Autodesk Inventor part; units mm, degrees
(part 2 of 2)
  spline S264 degree 2 poles (69.3218, -34.0148) (69.0307, -34.1828) (68.5047, -34.6064) (68.3514, -34.7463) knots 0 0 0 1 2 2 2
  line L285 (68.3514, -34.7463) -> (66.7794, -32.0236)
  line L286 (66.7794, -32.0236) -> (69.6777, -30.3503)
  line L287 (69.6777, -30.3503) -> (70.0361, -30.971)
  line L288 (70.0361, -30.971) -> (67.8185, -32.2513)
  line L289 (67.8185, -32.2513) -> (68.6317, -33.6598)
  spline S265 degree 2 poles (68.6317, -33.6598) (68.7502, -33.5685) (68.9911, -33.4123) (69.0938, -33.353) knots 0 0 0 1 2 2 2
  spline S266 degree 2 poles (69.0938, -33.353) (69.5005, -33.1182) (70.138, -32.9271) (70.5085, -32.9757) knots 0 0 0 1 2 2 2
  spline S267 degree 2 poles (70.5085, -32.9757) (70.8834, -33.0219) (71.5119, -33.4581) (71.7888, -33.9376) knots 0 0 0 1 2 2 2
  spline S268 degree 2 poles (75.2825, -30.6362) (76.103, -32.0575) (76.0455, -33.8659) (75.185, -34.3627) knots 0 0 0 1 2 2 2
  spline S269 degree 2 poles (75.185, -34.3627) (74.3117, -34.8669) (72.7105, -33.9819) (71.9072, -32.5906) knots 0 0 0 1 2 2 2
  spline S270 degree 2 poles (71.9072, -32.5906) (71.0817, -31.1607) (71.1442, -29.3609) (72.009, -28.8616) knots 0 0 0 1 2 2 2
  spline S271 degree 2 poles (72.009, -28.8616) (72.878, -28.3598) (74.4866, -29.2577) (75.2825, -30.6362) knots 0 0 0 1 2 2 2
  spline S272 degree 2 poles (75.3042, -32.7698) (75.2562, -32.4493) (74.8771, -31.5951) (74.5633, -31.0514) knots 0 0 0 1 2 2 2
  spline S273 degree 2 poles (74.5633, -31.0514) (74.2494, -30.5077) (73.7015, -29.7566) (73.4388, -29.5487) knots 0 0 0 1 2 2 2
  spline S274 degree 2 poles (73.4388, -29.5487) (73.1761, -29.3408) (72.643, -29.2775) (72.3476, -29.4481) knots 0 0 0 1 2 2 2
  spline S275 degree 2 poles (72.3476, -29.4481) (72.0522, -29.6186) (71.8318, -30.1169) (71.8812, -30.4594) knots 0 0 0 1 2 2 2
  spline S276 degree 2 poles (71.8812, -30.4594) (71.9299, -30.7909) (72.3274, -31.6573) (72.6264, -32.1753) knots 0 0 0 1 2 2 2
  spline S277 degree 2 poles (72.6264, -32.1753) (72.9477, -32.7319) (73.4463, -33.4372) (73.7257, -33.6641) knots 0 0 0 1 2 2 2
  spline S278 degree 2 poles (73.7257, -33.6641) (73.9866, -33.8787) (74.5382, -33.9541) (74.8464, -33.7762) knots 0 0 0 1 2 2 2
  spline S279 degree 2 poles (74.8464, -33.7762) (75.1375, -33.6081) (75.3579, -33.1099) (75.3042, -32.7698) knots 0 0 0 1 2 2 2
  spline S280 degree 2 poles (27.4559, -29.5461) (27.2633, -29.4349) (26.8279, -29.3091) (26.6018, -29.2756) knots 0 0 0 1 2 2 2
  spline S281 degree 2 poles (26.6018, -29.2756) (26.3885, -29.2495) (26.047, -29.2578) (25.909, -29.2695) knots 0 0 0 1 2 2 2
  line L290 (25.909, -29.2695) -> (25.8662, -29.2447)
  line L291 (25.8662, -29.2447) -> (26.2987, -28.4956)
  spline S282 degree 2 poles (26.2987, -28.4956) (26.6016, -28.5049) (27.5097, -28.7609) (27.865, -28.9661) knots 0 0 0 1 2 2 2
  spline S283 degree 2 poles (27.865, -28.9661) (28.2246, -29.1737) (28.6757, -29.6282) (28.8051, -29.9084) knots 0 0 0 1 2 2 2
  spline S284 degree 2 poles (28.8051, -29.9084) (28.9399, -30.2088) (28.9003, -30.831) (28.7124, -31.1563) knots 0 0 0 1 2 2 2
  spline S285 degree 2 poles (28.7124, -31.1563) (28.4603, -31.593) (27.5061, -31.9211) (27.0542, -31.7743) knots 0 0 0 1 2 2 2
  line L292 (27.0542, -31.7743) -> (27.0245, -31.8257)
  spline S286 degree 2 poles (27.0245, -31.8257) (27.1717, -31.9564) (27.4638, -32.3305) (27.5375, -32.5785) knots 0 0 0 1 2 2 2
  spline S287 degree 2 poles (27.5375, -32.5785) (27.6136, -32.8222) (27.5423, -33.4204) (27.3421, -33.7671) knots 0 0 0 1 2 2 2
  spline S288 degree 2 poles (27.3421, -33.7671) (27.137, -34.1224) (26.5444, -34.5852) (26.1884, -34.6878) knots 0 0 0 1 2 2 2
  spline S289 degree 2 poles (26.1884, -34.6878) (25.8188, -34.7941) (25.0204, -34.6642) (24.6052, -34.4245) knots 0 0 0 1 2 2 2
  spline S290 degree 2 poles (24.6052, -34.4245) (24.207, -34.1946) (23.5391, -33.5521) (23.3503, -33.2662) knots 0 0 0 1 2 2 2
  line L293 (23.3503, -33.2662) -> (23.7828, -32.517)
  line L294 (23.7828, -32.517) -> (23.8342, -32.5467)
  spline S291 degree 2 poles (23.8342, -32.5467) (23.9629, -32.8379) (24.5433, -33.5726) (24.9158, -33.7876) knots 0 0 0 1 2 2 2
  spline S292 degree 2 poles (24.9158, -33.7876) (25.1341, -33.9136) (25.6499, -34.0288) (25.8869, -33.9544) knots 0 0 0 1 2 2 2
  spline S293 degree 2 poles (25.8869, -33.9544) (26.1196, -33.8776) (26.4869, -33.5873) (26.6525, -33.3005) knots 0 0 0 1 2 2 2
  spline S294 degree 2 poles (26.6525, -33.3005) (26.8181, -33.0137) (26.8662, -32.5448) (26.7782, -32.3513) knots 0 0 0 1 2 2 2
  spline S295 degree 2 poles (26.7782, -32.3513) (26.6901, -32.1578) (26.3304, -31.8416) (26.0907, -31.7032) knots 0 0 0 1 2 2 2
  line L295 (26.0907, -31.7032) -> (25.791, -31.5302)
  line L296 (25.791, -31.5302) -> (26.1296, -30.9437)
  line L297 (26.1296, -30.9437) -> (26.3651, -31.0797)
  spline S296 degree 2 poles (26.3651, -31.0797) (26.8403, -31.354) (27.7016, -31.2462) (27.9512, -30.8139) knots 0 0 0 1 2 2 2
  spline S297 degree 2 poles (27.9512, -30.8139) (28.0674, -30.6127) (28.0789, -30.2369) (28.0042, -30.0796) knots 0 0 0 1 2 2 2
  spline S298 degree 2 poles (28.0042, -30.0796) (27.9234, -29.913) (27.64, -29.6524) (27.4559, -29.5461) knots 0 0 0 1 2 2 2
  spline S299 degree 2 poles (32.0466, -35.0505) (31.226, -36.4718) (29.6311, -37.3262) (28.7706, -36.8294) knots 0 0 0 1 2 2 2
  spline S300 degree 2 poles (28.7706, -36.8294) (27.8973, -36.3252) (27.8631, -34.496) (28.6664, -33.1047) knots 0 0 0 1 2 2 2
  spline S301 degree 2 poles (28.6664, -33.1047) (29.4919, -31.6748) (31.0819, -30.829) (31.9466, -31.3283) knots 0 0 0 1 2 2 2
  spline S302 degree 2 poles (31.9466, -31.3283) (32.8157, -31.83) (32.8424, -33.672) (32.0466, -35.0505) knots 0 0 0 1 2 2 2
  spline S303 degree 2 poles (30.2096, -36.1362) (30.4632, -35.9344) (31.0134, -35.179) (31.3273, -34.6353) knots 0 0 0 1 2 2 2
  spline S304 degree 2 poles (31.3273, -34.6353) (31.6412, -34.0916) (32.0178, -33.2416) (32.0665, -32.9101) knots 0 0 0 1 2 2 2
  spline S305 degree 2 poles (32.0665, -32.9101) (32.1152, -32.5786) (31.9034, -32.0853) (31.608, -31.9148) knots 0 0 0 1 2 2 2
  spline S306 degree 2 poles (31.608, -31.9148) (31.3126, -31.7443) (30.771, -31.8025) (30.499, -32.0165) knots 0 0 0 1 2 2 2
  spline S307 degree 2 poles (30.499, -32.0165) (30.2363, -32.2245) (29.6846, -33.0019) (29.3856, -33.5199) knots 0 0 0 1 2 2 2
  spline S308 degree 2 poles (29.3856, -33.5199) (29.0643, -34.0765) (28.7027, -34.8609) (28.6459, -35.2163) knots 0 0 0 1 2 2 2
  spline S309 degree 2 poles (28.6459, -35.2163) (28.5905, -35.5496) (28.801, -36.0649) (29.1092, -36.2429) knots 0 0 0 1 2 2 2
  spline S310 degree 2 poles (29.1092, -36.2429) (29.4003, -36.411) (29.942, -36.3527) (30.2096, -36.1362) knots 0 0 0 1 2 2 2
  spline S311 degree 2 poles (36.0108, -37.3393) (35.1902, -38.7606) (33.5953, -39.6149) (32.7348, -39.1181) knots 0 0 0 1 2 2 2
  spline S312 degree 2 poles (32.7348, -39.1181) (31.8615, -38.6139) (31.8273, -36.7848) (32.6306, -35.3934) knots 0 0 0 1 2 2 2
  spline S313 degree 2 poles (32.6306, -35.3934) (33.4561, -33.9636) (35.0461, -33.1178) (35.9108, -33.617) knots 0 0 0 1 2 2 2
  spline S314 degree 2 poles (35.9108, -33.617) (36.7799, -34.1188) (36.8066, -35.9608) (36.0108, -37.3393) knots 0 0 0 1 2 2 2
  spline S315 degree 2 poles (34.1739, -38.4249) (34.4274, -38.2231) (34.9777, -37.4677) (35.2916, -36.924) knots 0 0 0 1 2 2 2
  spline S316 degree 2 poles (35.2916, -36.924) (35.6054, -36.3803) (35.982, -35.5304) (36.0307, -35.1989) knots 0 0 0 1 2 2 2
  spline S317 degree 2 poles (36.0307, -35.1989) (36.0794, -34.8674) (35.8676, -34.3741) (35.5722, -34.2035) knots 0 0 0 1 2 2 2
  spline S318 degree 2 poles (35.5722, -34.2035) (35.2768, -34.033) (34.7352, -34.0913) (34.4632, -34.3053) knots 0 0 0 1 2 2 2
  spline S319 degree 2 poles (34.4632, -34.3053) (34.2005, -34.5132) (33.6489, -35.2907) (33.3498, -35.8087) knots 0 0 0 1 2 2 2
  spline S320 degree 2 poles (33.3498, -35.8087) (33.0285, -36.3652) (32.6669, -37.1496) (32.6101, -37.505) knots 0 0 0 1 2 2 2
  spline S321 degree 2 poles (32.6101, -37.505) (32.5547, -37.8383) (32.7652, -38.3537) (33.0734, -38.5316) knots 0 0 0 1 2 2 2
  spline S322 degree 2 poles (33.0734, -38.5316) (33.3645, -38.6997) (33.9062, -38.6414) (34.1739, -38.4249) knots 0 0 0 1 2 2 2
  line L298 (19.7742, -20.8876) -> (21.6551, -24.1454)
  line L299 (21.6551, -24.1454) -> (20.9059, -24.5779)
  spline S323 degree 2 poles (20.9059, -24.5779) (20.3736, -24.4172) (19.4006, -24.1456) (18.8979, -24.0363) knots 0 0 0 1 2 2 2
  spline S324 degree 2 poles (18.8979, -24.0363) (17.8859, -23.8158) (16.835, -23.8345) (16.4112, -24.0792) knots 0 0 0 1 2 2 2
  spline S325 degree 2 poles (16.4112, -24.0792) (16.1886, -24.2078) (15.9338, -24.5375) (15.8984, -24.7235) knots 0 0 0 1 2 2 2
  spline S326 degree 2 poles (15.8984, -24.7235) (15.8631, -24.9094) (15.9439, -25.2966) (16.0576, -25.4935) knots 0 0 0 1 2 2 2
  spline S327 degree 2 poles (16.0576, -25.4935) (16.1663, -25.6819) (16.483, -26.0128) (16.6571, -26.1463) knots 0 0 0 1 2 2 2
  spline S328 degree 2 poles (16.6571, -26.1463) (16.8035, -26.2615) (17.1354, -26.4409) (17.2448, -26.4919) knots 0 0 0 1 2 2 2
  line L300 (17.2448, -26.4919) -> (17.267, -26.5304)
  line L301 (17.267, -26.5304) -> (16.5136, -26.9655)
  spline S329 degree 2 poles (16.5136, -26.9655) (16.2805, -26.8089) (15.6184, -26.1466) (15.4157, -25.7956) knots 0 0 0 1 2 2 2
  spline S330 degree 2 poles (15.4157, -25.7956) (14.9881, -25.0549) (15.2896, -23.7678) (15.9574, -23.3823) knots 0 0 0 1 2 2 2
  spline S331 degree 2 poles (15.9574, -23.3823) (16.2699, -23.2018) (16.8763, -23.0459) (17.173, -23.0458) knots 0 0 0 1 2 2 2
  spline S332 degree 2 poles (17.173, -23.0458) (17.4783, -23.0407) (18.1472, -23.1512) (18.4841, -23.2306) knots 0 0 0 1 2 2 2
  spline S333 degree 2 poles (18.4841, -23.2306) (19.0408, -23.3544) (20.292, -23.7223) (20.6598, -23.8353) knots 0 0 0 1 2 2 2
  line L302 (20.6598, -23.8353) -> (19.162, -21.241)
  line L303 (19.162, -21.241) -> (19.7742, -20.8876)
  line L304 (15.5887, -17.8301) -> (15.9521, -18.4594)
  line L305 (15.9521, -18.4594) -> (17.7672, -17.4114)
  line L306 (17.7672, -17.4114) -> (18.1602, -18.0921)
  line L307 (18.1602, -18.0921) -> (16.345, -19.14)
  line L308 (16.345, -19.14) -> (17.6921, -21.4732)
  line L309 (17.6921, -21.4732) -> (16.9472, -21.9032)
  line L310 (16.9472, -21.9032) -> (12.8601, -21.1121)
  line L311 (12.8601, -21.1121) -> (12.4844, -20.4614)
  line L312 (12.4844, -20.4614) -> (15.3827, -18.7881)
  line L313 (15.3827, -18.7881) -> (15.0194, -18.1588)
  line L314 (15.0194, -18.1588) -> (15.5887, -17.8301)
  line L315 (15.7757, -19.4688) -> (13.7122, -20.6601)
  line L316 (13.7122, -20.6601) -> (16.8014, -21.2454)
  line L317 (16.8014, -21.2454) -> (15.7757, -19.4688)
  spline S334 degree 2 poles (12.538, -14.4542) (13.9593, -13.6336) (15.7677, -13.6911) (16.2645, -14.5516) knots 0 0 0 1 2 2 2
  spline S335 degree 2 poles (16.2645, -14.5516) (16.7687, -15.425) (15.8838, -17.0261) (14.4924, -17.8294) knots 0 0 0 1 2 2 2
  spline S336 degree 2 poles (14.4924, -17.8294) (13.0626, -18.6549) (11.2627, -18.5924) (10.7634, -17.7277) knots 0 0 0 1 2 2 2
  spline S337 degree 2 poles (10.7634, -17.7277) (10.2617, -16.8586) (11.1595, -15.25) (12.538, -14.4542) knots 0 0 0 1 2 2 2
  spline S338 degree 2 poles (14.6717, -14.4324) (14.3512, -14.4804) (13.4969, -14.8595) (12.9533, -15.1734) knots 0 0 0 1 2 2 2
  spline S339 degree 2 poles (12.9533, -15.1734) (12.4096, -15.4873) (11.6585, -16.0351) (11.4505, -16.2978) knots 0 0 0 1 2 2 2
  spline S340 degree 2 poles (11.4505, -16.2978) (11.2426, -16.5606) (11.1794, -17.0937) (11.3499, -17.3891) knots 0 0 0 1 2 2 2
  spline S341 degree 2 poles (11.3499, -17.3891) (11.5205, -17.6845) (12.0187, -17.9048) (12.3613, -17.8555) knots 0 0 0 1 2 2 2
  spline S342 degree 2 poles (12.3613, -17.8555) (12.6927, -17.8068) (13.5592, -17.4093) (14.0772, -17.1102) knots 0 0 0 1 2 2 2
  spline S343 degree 2 poles (14.0772, -17.1102) (14.6337, -16.7889) (15.3391, -16.2903) (15.5659, -16.011) knots 0 0 0 1 2 2 2
  spline S344 degree 2 poles (15.5659, -16.011) (15.7806, -15.75) (15.856, -15.1985) (15.678, -14.8902) knots 0 0 0 1 2 2 2
  spline S345 degree 2 poles (15.678, -14.8902) (15.51, -14.5991) (15.0117, -14.3788) (14.6717, -14.4324) knots 0 0 0 1 2 2 2
  line L318 (13.5615, -2.8735) -> (13.5615, -6.6353)
  line L319 (13.5615, -6.6353) -> (12.6964, -6.6353)
  spline S346 degree 2 poles (12.6964, -6.6353) (12.3158, -6.23) (11.6089, -5.5083) (11.2283, -5.1623) knots 0 0 0 1 2 2 2
  spline S347 degree 2 poles (11.2283, -5.1623) (10.4621, -4.4652) (9.5426, -3.9561) (9.0532, -3.9561) knots 0 0 0 1 2 2 2
  spline S348 degree 2 poles (9.0532, -3.9561) (8.7962, -3.9561) (8.4106, -4.1143) (8.287, -4.2576) knots 0 0 0 1 2 2 2
  spline S349 degree 2 poles (8.287, -4.2576) (8.1634, -4.401) (8.0398, -4.7767) (8.0398, -5.0041) knots 0 0 0 1 2 2 2
  spline S350 degree 2 poles (8.0398, -5.0041) (8.0398, -5.2216) (8.1486, -5.6665) (8.2326, -5.8691) knots 0 0 0 1 2 2 2
  spline S351 degree 2 poles (8.2326, -5.8691) (8.3018, -6.0422) (8.4996, -6.3635) (8.5688, -6.4623) knots 0 0 0 1 2 2 2
  line L320 (8.5688, -6.4623) -> (8.5688, -6.5068)
  line L321 (8.5688, -6.5068) -> (7.6988, -6.5068)
  spline S352 degree 2 poles (7.6988, -6.5068) (7.5752, -6.2547) (7.333, -5.3501) (7.333, -4.9447) knots 0 0 0 1 2 2 2
  spline S353 degree 2 poles (7.333, -4.9447) (7.333, -4.0896) (8.2376, -3.1256) (9.0087, -3.1256) knots 0 0 0 1 2 2 2
  spline S354 degree 2 poles (9.0087, -3.1256) (9.3696, -3.1256) (9.9727, -3.2937) (10.2297, -3.442) knots 0 0 0 1 2 2 2
  spline S355 degree 2 poles (10.2297, -3.442) (10.4967, -3.5903) (11.0206, -4.0204) (11.2727, -4.2576) knots 0 0 0 1 2 2 2
  spline S356 degree 2 poles (11.2727, -4.2576) (11.6929, -4.6432) (12.5926, -5.5874) (12.8546, -5.8691) knots 0 0 0 1 2 2 2
  line L322 (12.8546, -5.8691) -> (12.8546, -2.8735)
  line L323 (12.8546, -2.8735) -> (13.5615, -2.8735)
  line L324 (8.376, 1.7732) -> (13.5615, -0.8665)
  line L325 (13.5615, -0.8665) -> (13.5615, -1.7366)
  line L326 (13.5615, -1.7366) -> (8.1783, 1.0514)
  line L327 (8.1783, 1.0514) -> (8.1783, -2.0974)
  line L328 (8.1783, -2.0974) -> (7.4615, -2.0974)
  line L329 (7.4615, -2.0974) -> (7.4615, 1.7732)
  line L330 (7.4615, 1.7732) -> (8.376, 1.7732)
  spline S357 degree 2 poles (10.5115, 6.316) (12.1527, 6.316) (13.69, 5.362) (13.69, 4.3684) knots 0 0 0 1 2 2 2
  spline S358 degree 2 poles (13.69, 4.3684) (13.69, 3.36) (12.123, 2.4158) (10.5164, 2.4158) knots 0 0 0 1 2 2 2
  spline S359 degree 2 poles (10.5164, 2.4158) (8.8654, 2.4158) (7.3379, 3.3698) (7.3379, 4.3684) knots 0 0 0 1 2 2 2
  spline S360 degree 2 poles (7.3379, 4.3684) (7.3379, 5.3719) (8.9198, 6.316) (10.5115, 6.316) knots 0 0 0 1 2 2 2
  spline S361 degree 2 poles (12.3702, 5.2681) (12.0686, 5.3867) (11.1393, 5.4856) (10.5115, 5.4856) knots 0 0 0 1 2 2 2
  spline S362 degree 2 poles (10.5115, 5.4856) (9.8837, 5.4856) (8.9593, 5.3867) (8.6479, 5.2631) knots 0 0 0 1 2 2 2
  spline S363 degree 2 poles (8.6479, 5.2631) (8.3364, 5.1395) (8.0151, 4.7095) (8.0151, 4.3684) knots 0 0 0 1 2 2 2
  spline S364 degree 2 poles (8.0151, 4.3684) (8.0151, 4.0273) (8.3364, 3.5873) (8.6578, 3.4588) knots 0 0 0 1 2 2 2
  spline S365 degree 2 poles (8.6578, 3.4588) (8.9692, 3.3352) (9.9183, 3.2463) (10.5164, 3.2463) knots 0 0 0 1 2 2 2
  spline S366 degree 2 poles (10.5164, 3.2463) (11.1591, 3.2463) (12.0192, 3.3254) (12.3553, 3.4539) knots 0 0 0 1 2 2 2
  spline S367 degree 2 poles (12.3553, 3.4539) (12.6717, 3.5725) (13.0128, 4.0125) (13.0128, 4.3684) knots 0 0 0 1 2 2 2
  spline S368 degree 2 poles (13.0128, 4.3684) (13.0128, 4.7045) (12.6915, 5.1445) (12.3702, 5.2681) knots 0 0 0 1 2 2 2
  point P0 (0, 0)
  point P1 (97.5334, -46.673)
  point P2 (50, 21.5)
  point P3 (50, 35)
  point P4 (85.5155, 4.3292)
  point P5 (43.9223, 34.4683)
  point P6 (38.0293, 32.8892)
  point P7 (32.5, 30.3109)
  point P8 (27.5024, 26.8116)
  point P9 (23.1884, 22.4976)
  point P10 (19.6891, 17.5)
  point P11 (17.1108, 11.9707)
  point P12 (15.5317, 6.0777)
  point P13 (15, 0)
  point P14 (15.5317, -6.0777)
  point P15 (17.1108, -11.9707)
  point P16 (19.6891, -17.5)
  point P17 (23.1884, -22.4976)
  point P18 (27.5024, -26.8116)
  point P19 (32.5, -30.3109)
  point P20 (38.0293, -32.8892)
  point P21 (43.9223, -34.4683)
  point P22 (50, -35)
  point P23 (56.0777, -34.4683)
  point P24 (61.9707, -32.8892)
  point P25 (67.5, -30.3109)
  point P26 (72.4976, -26.8116)
  point P27 (76.8116, -22.4976)
  point P28 (80.3109, -17.5)
  point P29 (82.8892, -11.9707)
  point P30 (84.4683, -6.0777)
  point P31 (85, 0)
  point P32 (84.4683, 6.0777)
  point P33 (82.8892, 11.9707)
  point P34 (80.3109, 17.5)
  point P35 (76.8116, 22.4976)
  point P36 (72.4976, 26.8116)
  point P37 (67.5, 30.3109)
  point P38 (61.9707, 32.8892)
  point P39 (56.0777, 34.4683)
  point P40 (0, 15)
  point P41 (0, -15)
  point P42 (72.5, 38.9711)
  point P43 (72.5, -38.9711)
  point P44 (27.5, 38.9711)
  point P45 (27.5, -38.9711)
  point P46 (12.5, 24.8747)
  point P47 (12.5, -24.8747)
  dimension "d3" = 12
  dimension "d4" = 25
  dimension "d5" = 20.96
  dimension "d6" = 15.75
  dimension "d7" = 50
  dimension "d8" = 2.5
  dimension "d9" = 7
  dimension "d10" = 21.5
  dimension "d11" = 2.5
  dimension "d12" = 3
  dimension "d14" = 5
  dimension "d15" = 2
  dimension "d16" = 30
  dimension "d27" = 360
  dimension "d32" = 45
  dimension "d33" = 3
  dimension "d44" = 55
  dimension "d51" = 14.5786
  dimension "d52" = 14.5786
  dimension "d53" = 14.5786
  constraints: 320 end point, 30 point on circle, 20 centre point, 14 parallel, 8 point on line, 8 tangent, 7 equal radius, 6 midpoint, 6 perpendicular, 4 coincident, 4 horizontal, 2 concentric, 1 vertical, 360 other
  measures "d3" diameter of A0
  measures "d4" diameter of A1
  measures "d5" distance of A5.centre A4.centre
  measures "d6" distance from line of L1 A4.centre
  measures "d7" distance from line of L0 A0.centre
  measures "d8" radius of A3
  measures "d9" distance of L2.start L2.end
  measures "d10" distance from line of L1 L2.start
  measures "d11" diameter of A4
  measures "d12" diameter of A7
  measures "d14" distance of L12.end L10.start
  measures "d15" distance of L10.start L10.end
  measures "d16" distance from line of A0.centre L12
  measures "d32" radius of A11
  measures "d33" diameter of A13
  measures "d44" distance of L171.start L171.end
  measures "d51" distance of L189.end L190.end
  measures "d52" distance of L194.end L195.end
  measures "d53" distance of L198.end L199.end
extrude "Extrusion1" add sketch "Sketch1" against normal blind 4 contours L13 L12 L11 L10 | L34 L33 L32 L31 | L38 L37 L36 L35 | L42 L41 L40 L39 | L46 L45 L176 L43 | L43 L176 A19 S127 S126 S125 S124 S123 S122 S121 S120 A10 A18 S190 S189 S188 S187 L175 L157 L158 L155 L117 L118 L115 A16 S270 S269 S268 A11 A17 S290 S289 S288 S287 S286 L292 S285 S284 S283 L85 L86 L83 L45 L46 | L176 L45 L44 L43 | L43 L44 L45 L176 L83 L84 L85 A17 S283 S282 L291 L290 S281 S280 S298 S297 S296 L297 L296 L295 S295 S291 L294 L293 S290 A11 A10 A19 S120 L232 L231 S119 S118 S134 L238 L237 L236 S133 S132 S131 S130 S129 L235 L234 S128 S127 | S127 S128 L234 L235 S129 S130 S131 S132 S133 L236 L237 L238 S134 A19 S123 L233 S124 | A19 S124 S125 S126 S127 | L176 L85 L84 L83 | L83 L86 L85 L176 | S124 L233 S123 A19 | A19 S134 S135 S136 S118 S120 S121 S122 S123 | A19 S118 S136 S135 S134 | S283 S284 S285 L292 S286 S287 S288 S289 S290 A17 S291 S292 S293 S294 S295 S296 S297 | A17 S297 S298 S280 S281 L290 L291 S282 S283 | S118 S119 L231 L232 S120 A19 | S297 S296 A17 | A17 S295 L295 L296 L297 S296 | S295 S294 S293 S292 S291 A17 | A10 A11 A16 S268 S271 S270 L175 L115 L116 L117 L155 L156 L157 A18 S187 S190 | A17 S290 L293 L294 S291 | S190 S187 A18 S191 | A18 S191 S192 S193 S194 S195 S196 S197 S198 S187 S188 S189 S190 | S191 A18 | A18 S191 S198 S197 S196 S195 S194 S193 S192 | S268 S269 S270 A16 S275 S276 S277 S278 S279 | A16 S279 S272 S273 S274 S275 S270 S271 S268 | S279 S278 S277 S276 S275 A16 | A16 S275 S274 S273 S272 S279 | L175 L155 L158 L157 | L157 L156 L155 L175 | L175 L115 L118 L117 | L117 L116 L115 L175 | L50 L49 L48 L47 | L54 L53 L52 L51 | L58 L57 L56 L55 | L62 L61 L60 L59 | L66 L65 L64 L63 | L70 L69 L68 L67 | L74 L73 L72 L71 | L78 L77 L76 L75 | L82 L81 L80 L79 | L90 L89 L88 L87 | L94 L93 L92 L91 | L98 L97 L96 L95 | L102 L101 L100 L99 | L106 L105 L104 L103 | L110 L109 L108 L107 | L114 L113 L112 L111 | L122 L121 L120 L119 | L126 L125 L124 L123 | L130 L129 L128 L127 | L134 L133 L132 L131 | L138 L137 L136 L135 | L142 L141 L140 L139 | L146 L145 L144 L143 | L150 L149 L148 L147 | L154 L153 L152 L151 | L162 L161 L160 L159 | L166 L165 L164 L163 | L170 L169 L168 L167 | S0 S1 L209 L210 S2 S3 S4 S5 L211 S6 S7 S8 S9 S10 L212 L213 S11 S12 S13 S14 S15 L214 L215 L216 S16 S17 S18 | S19 S20 S21 S22 | S30 S29 S28 S27 S26 S25 S24 S23 | S31 S32 S33 S34 | S42 S41 S40 S39 S38 S37 S36 S35 | L217 L218 L219 L220 L221 L222 S43 L223 L224 L225 L226 | S44 S45 S46 L227 S47 S48 S49 S50 L228 S51 S52 | S57 S56 S55 S54 S53 | S62 S61 S60 S59 S58 | S63 S64 S65 S66 | S74 S73 S72 S71 S70 S69 S68 S67 | S75 S76 S77 S78 S79 S80 S81 L229 L230 S82 S83 S84 S85 S86 | S93 S92 S91 S90 S89 S88 S87 | S94 S95 S96 S97 | S105 S104 S103 S102 S101 S100 S99 S98 | S106 S107 S108 S109 | S117 S116 S115 S114 S113 S112 S111 S110 | S137 S138 L239 L240 S139 S140 S141 S142 L241 S143 S144 S145 S146 S147 L242 L243 S148 S149 S150 S151 S152 L244 L245 L246 S153 S154 S155 | S156 S157 S158 S159 | S167 S166 S165 S164 S163 S162 S161 S160 | S168 S169 L247 L248 S170 S171 S172 S173 L249 S174 S175 S176 S177 S178 L250 L251 S179 S180 S181 S182 S183 L252 L253 L254 S184 S185 S186 | S199 S200 S201 S202 S203 S204 S205 L255 L256 S206 S207 S208 S209 S210 | S217 S216 S215 S214 S213 S212 S211 | S218 S219 S220 S221 | S229 S228 S227 S226 S225 S224 S223 S222 | L257 L258 L259 L260 L261 L262 S230 L263 L264 L265 L266 | L267 L268 S231 S232 S233 S234 S235 S236 L269 L270 S237 S238 S239 S240 S241 L271 L272 | S242 S243 S244 S245 | S253 S252 S251 S250 S249 S248 S247 S246 | L273 L274 L275 L276 L277 L278 S254 L279 L280 L281 L282 | S255 S256 S257 L283 L284 S258 S259 S260 S261 S262 S263 S264 L285 L286 L287 L288 L289 S265 S266 S267 | S299 S300 S301 S302 | S310 S309 S308 S307 S306 S305 S304 S303 | S311 S312 S313 S314 | S322 S321 S320 S319 S318 S317 S316 S315 | L298 L299 S323 S324 S325 S326 S327 S328 L300 L301 S329 S330 S331 S332 S333 L302 L303 | L304 L305 L306 L307 L308 L309 L310 L311 L312 L313 L314 | L317 L316 L315 | S334 S335 S336 S337 | S345 S344 S343 S342 S341 S340 S339 S338 | L318 L319 S346 S347 S348 S349 S350 S351 L320 L321 S352 S353 S354 S355 S356 L322 L323 | L324 L325 L326 L327 L328 L329 L330 | S357 S358 S359 S360 | S368 S367 S366 S365 S364 S363 S362 S361
extrude "Extrusion2" add sketch "Sketch1" along normal blind 1.5 contours L13 L12 L11 L10 | L34 L33 L32 L31 | L38 L37 L36 L35 | L42 L41 L40 L39 | L46 L45 L176 L43 | L176 L45 L44 L43 | L176 L85 L84 L83 | L83 L86 L85 L176 | L175 L155 L158 L157 | L157 L156 L155 L175 | L175 L115 L118 L117 | L117 L116 L115 L175 | L50 L49 L48 L47 | L54 L53 L52 L51 | L58 L57 L56 L55 | L62 L61 L60 L59 | L66 L65 L64 L63 | L70 L69 L68 L67 | L74 L73 L72 L71 | L78 L77 L76 L75 | L82 L81 L80 L79 | L90 L89 L88 L87 | L94 L93 L92 L91 | L98 L97 L96 L95 | L102 L101 L100 L99 | L106 L105 L104 L103 | L110 L109 L108 L107 | L114 L113 L112 L111 | L122 L121 L120 L119 | L126 L125 L124 L123 | L130 L129 L128 L127 | L134 L133 L132 L131 | L138 L137 L136 L135 | L142 L141 L140 L139 | L146 L145 L144 L143 | L150 L149 L148 L147 | L154 L153 L152 L151 | L162 L161 L160 L159 | L166 L165 L164 L163 | L170 L169 L168 L167
extrude "Extrusion3" add sketch "Sketch1" along normal blind 1 contours S127 S128 L234 L235 S129 S130 S131 S132 S133 L236 L237 L238 S134 A19 S123 L233 S124 | A19 S124 S125 S126 S127 | A19 S134 S135 S136 S118 S120 S121 S122 S123 | S283 S284 S285 L292 S286 S287 S288 S289 S290 A17 S291 S292 S293 S294 S295 S296 S297 | A17 S297 S298 S280 S281 L290 L291 S282 S283 | S118 S119 L231 L232 S120 A19 | A17 S295 L295 L296 L297 S296 | A17 S290 L293 L294 S291 | S190 S187 A18 S191 | A18 S191 S192 S193 S194 S195 S196 S197 S198 S187 S188 S189 S190 | S268 S269 S270 A16 S275 S276 S277 S278 S279 | A16 S279 S272 S273 S274 S275 S270 S271 S268 | S0 S1 L209 L210 S2 S3 S4 S5 L211 S6 S7 S8 S9 S10 L212 L213 S11 S12 S13 S14 S15 L214 L215 L216 S16 S17 S18 | S19 S20 S21 S22 | S31 S32 S33 S34 | L217 L218 L219 L220 L221 L222 S43 L223 L224 L225 L226 | S44 S45 S46 L227 S47 S48 S49 S50 L228 S51 S52 | S63 S64 S65 S66 | S75 S76 S77 S78 S79 S80 S81 L229 L230 S82 S83 S84 S85 S86 | S94 S95 S96 S97 | S106 S107 S108 S109 | S137 S138 L239 L240 S139 S140 S141 S142 L241 S143 S144 S145 S146 S147 L242 L243 S148 S149 S150 S151 S152 L244 L245 L246 S153 S154 S155 | S156 S157 S158 S159 | S168 S169 L247 L248 S170 S171 S172 S173 L249 S174 S175 S176 S177 S178 L250 L251 S179 S180 S181 S182 S183 L252 L253 L254 S184 S185 S186 | S199 S200 S201 S202 S203 S204 S205 L255 L256 S206 S207 S208 S209 S210 | S218 S219 S220 S221 | L257 L258 L259 L260 L261 L262 S230 L263 L264 L265 L266 | L267 L268 S231 S232 S233 S234 S235 S236 L269 L270 S237 S238 S239 S240 S241 L271 L272 | S242 S243 S244 S245 | L273 L274 L275 L276 L277 L278 S254 L279 L280 L281 L282 | S255 S256 S257 L283 L284 S258 S259 S260 S261 S262 S263 S264 L285 L286 L287 L288 L289 S265 S266 S267 | S299 S300 S301 S302 | S311 S312 S313 S314 | L298 L299 S323 S324 S325 S326 S327 S328 L300 L301 S329 S330 S331 S332 S333 L302 L303 | L304 L305 L306 L307 L308 L309 L310 L311 L312 L313 L314 | S334 S335 S336 S337 | L318 L319 S346 S347 S348 S349 S350 S351 L320 L321 S352 S353 S354 S355 S356 L322 L323 | L324 L325 L326 L327 L328 L329 L330 | S357 S358 S359 S360
extrude "Extrusion4" add sketch "Sketch1" against normal blind 20 from surface at -4 separate body contours L176 L45 L44 L43 | L43 L44 L45 L176 L83 L84 L85 A17 S283 S282 L291 L290 S281 S280 S298 S297 S296 L297 L296 L295 S295 S291 L294 L293 S290 A11 A10 A19 S120 L232 L231 S119 S118 S134 L238 L237 L236 S133 S132 S131 S130 S129 L235 L234 S128 S127 | S127 S128 L234 L235 S129 S130 S131 S132 S133 L236 L237 L238 S134 A19 S123 L233 S124 | L176 L85 L84 L83 | S124 L233 S123 A19 | A17 S297 S298 S280 S281 L290 L291 S282 S283 | S118 S119 L231 L232 S120 A19 | A17 S295 L295 L296 L297 S296 | A10 A11 A16 S268 S271 S270 L175 L115 L116 L117 L155 L156 L157 A18 S187 S190 | A17 S290 L293 L294 S291 | S190 S187 A18 S191 | S191 A18 | A16 S279 S272 S273 S274 S275 S270 S271 S268 | A16 S275 S274 S273 S272 S279 | L157 L156 L155 L175 | L117 L116 L115 L175 | L50 L49 L48 L47 | L54 L53 L52 L51 | L58 L57 L56 L55 | L62 L61 L60 L59 | L66 L65 L64 L63 | L70 L69 L68 L67 | L74 L73 L72 L71 | L78 L77 L76 L75 | L82 L81 L80 L79 | L122 L121 L120 L119 | L126 L125 L124 L123 | L130 L129 L128 L127 | L134 L133 L132 L131 | L138 L137 L136 L135 | L142 L141 L140 L139 | L146 L145 L144 L143 | L150 L149 L148 L147 | L154 L153 L152 L151 | S0 S1 L209 L210 S2 S3 S4 S5 L211 S6 S7 S8 S9 S10 L212 L213 S11 S12 S13 S14 S15 L214 L215 L216 S16 S17 S18 | S19 S20 S21 S22 | S30 S29 S28 S27 S26 S25 S24 S23 | S31 S32 S33 S34 | S42 S41 S40 S39 S38 S37 S36 S35 | S75 S76 S77 S78 S79 S80 S81 L229 L230 S82 S83 S84 S85 S86 | S93 S92 S91 S90 S89 S88 S87 | S94 S95 S96 S97 | S105 S104 S103 S102 S101 S100 S99 S98 | S199 S200 S201 S202 S203 S204 S205 L255 L256 S206 S207 S208 S209 S210 | S217 S216 S215 S214 S213 S212 S211 | S218 S219 S220 S221 | S229 S228 S227 S226 S225 S224 S223 S222 | L257 L258 L259 L260 L261 L262 S230 L263 L264 L265 L266 | L267 L268 S231 S232 S233 S234 S235 S236 L269 L270 S237 S238 S239 S240 S241 L271 L272 | S242 S243 S244 S245 | S253 S252 S251 S250 S249 S248 S247 S246 | L298 L299 S323 S324 S325 S326 S327 S328 L300 L301 S329 S330 S331 S332 S333 L302 L303 | L304 L305 L306 L307 L308 L309 L310 L311 L312 L313 L314 | L317 L316 L315 | S334 S335 S336 S337 | S345 S344 S343 S342 S341 S340 S339 S338 | L318 L319 S346 S347 S348 S349 S350 S351 L320 L321 S352 S353 S354 S355 S356 L322 L323 | L324 L325 L326 L327 L328 L329 L330 | S357 S358 S359 S360 | S368 S367 S366 S365 S364 S363 S362 S361
extrude "Extrusion5" add sketch "Sketch1" against normal blind 3 from surface at -24 contours A0 | A2 L4 A3 L3 | A4 | A5 | A6 | A7 | A8 | A9 | L13 L12 L11 L10 | L34 L33 L32 L31 | L38 L37 L36 L35 | L42 L41 L40 L39 | L46 L45 L176 L43 | L43 L176 A19 S127 S126 S125 S124 S123 S122 S121 S120 A10 A18 S190 S189 S188 S187 L175 L157 L158 L155 L117 L118 L115 A16 S270 S269 S268 A11 A17 S290 S289 S288 S287 S286 L292 S285 S284 S283 L85 L86 L83 L45 L46 | L176 L45 L44 L43 | L43 L44 L45 L176 L83 L84 L85 A17 S283 S282 L291 L290 S281 S280 S298 S297 S296 L297 L296 L295 S295 S291 L294 L293 S290 A11 A10 A19 S120 L232 L231 S119 S118 S134 L238 L237 L236 S133 S132 S131 S130 S129 L235 L234 S128 S127 | S127 S128 L234 L235 S129 S130 S131 S132 S133 L236 L237 L238 S134 A19 S123 L233 S124 | A19 S124 S125 S126 S127 | L176 L85 L84 L83 | L83 L86 L85 L176 | S124 L233 S123 A19 | A19 S134 S135 S136 S118 S120 S121 S122 S123 | A19 S118 S136 S135 S134 | S283 S284 S285 L292 S286 S287 S288 S289 S290 A17 S291 S292 S293 S294 S295 S296 S297 | A17 S297 S298 S280 S281 L290 L291 S282 S283 | S118 S119 L231 L232 S120 A19 | S297 S296 A17 | A17 S295 L295 L296 L297 S296 | S295 S294 S293 S292 S291 A17 | A10 A11 A16 S268 S271 S270 L175 L115 L116 L117 L155 L156 L157 A18 S187 S190 | A17 S290 L293 L294 S291 | S190 S187 A18 S191 | A18 S191 S192 S193 S194 S195 S196 S197 S198 S187 S188 S189 S190 | S191 A18 | A18 S191 S198 S197 S196 S195 S194 S193 S192 | S268 S269 S270 A16 S275 S276 S277 S278 S279 | A16 S279 S272 S273 S274 S275 S270 S271 S268 | S279 S278 S277 S276 S275 A16 | A16 S275 S274 S273 S272 S279 | L175 L155 L158 L157 | L157 L156 L155 L175 | L175 L115 L118 L117 | L117 L116 L115 L175 | L50 L49 L48 L47 | L54 L53 L52 L51 | L58 L57 L56 L55 | L62 L61 L60 L59 | L66 L65 L64 L63 | L70 L69 L68 L67 | L74 L73 L72 L71 | L78 L77 L76 L75 | L82 L81 L80 L79 | L90 L89 L88 L87 | L94 L93 L92 L91 | L98 L97 L96 L95 | L102 L101 L100 L99 | L106 L105 L104 L103 | L110 L109 L108 L107 | L114 L113 L112 L111 | L122 L121 L120 L119 | L126 L125 L124 L123 | L130 L129 L128 L127 | L134 L133 L132 L131 | L138 L137 L136 L135 | L142 L141 L140 L139 | L146 L145 L144 L143 | L150 L149 L148 L147 | L154 L153 L152 L151 | L162 L161 L160 L159 | L166 L165 L164 L163 | L170 L169 L168 L167 | S0 S1 L209 L210 S2 S3 S4 S5 L211 S6 S7 S8 S9 S10 L212 L213 S11 S12 S13 S14 S15 L214 L215 L216 S16 S17 S18 | S19 S20 S21 S22 | S30 S29 S28 S27 S26 S25 S24 S23 | S31 S32 S33 S34 | S42 S41 S40 S39 S38 S37 S36 S35 | L217 L218 L219 L220 L221 L222 S43 L223 L224 L225 L226 | S44 S45 S46 L227 S47 S48 S49 S50 L228 S51 S52 | S57 S56 S55 S54 S53 | S62 S61 S60 S59 S58 | S63 S64 S65 S66 | S74 S73 S72 S71 S70 S69 S68 S67 | S75 S76 S77 S78 S79 S80 S81 L229 L230 S82 S83 S84 S85 S86 | S93 S92 S91 S90 S89 S88 S87 | S94 S95 S96 S97 | S105 S104 S103 S102 S101 S100 S99 S98 | S106 S107 S108 S109 | S117 S116 S115 S114 S113 S112 S111 S110 | S137 S138 L239 L240 S139 S140 S141 S142 L241 S143 S144 S145 S146 S147 L242 L243 S148 S149 S150 S151 S152 L244 L245 L246 S153 S154 S155 | S156 S157 S158 S159 | S167 S166 S165 S164 S163 S162 S161 S160 | S168 S169 L247 L248 S170 S171 S172 S173 L249 S174 S175 S176 S177 S178 L250 L251 S179 S180 S181 S182 S183 L252 L253 L254 S184 S185 S186 | S199 S200 S201 S202 S203 S204 S205 L255 L256 S206 S207 S208 S209 S210 | S217 S216 S215 S214 S213 S212 S211 | S218 S219 S220 S221 | S229 S228 S227 S226 S225 S224 S223 S222 | L257 L258 L259 L260 L261 L262 S230 L263 L264 L265 L266 | L267 L268 S231 S232 S233 S234 S235 S236 L269 L270 S237 S238 S239 S240 S241 L271 L272 | S242 S243 S244 S245 | S253 S252 S251 S250 S249 S248 S247 S246 | L273 L274 L275 L276 L277 L278 S254 L279 L280 L281 L282 | S255 S256 S257 L283 L284 S258 S259 S260 S261 S262 S263 S264 L285 L286 L287 L288 L289 S265 S266 S267 | S299 S300 S301 S302 | S310 S309 S308 S307 S306 S305 S304 S303 | S311 S312 S313 S314 | S322 S321 S320 S319 S318 S317 S316 S315 | L298 L299 S323 S324 S325 S326 S327 S328 L300 L301 S329 S330 S331 S332 S333 L302 L303 | L304 L305 L306 L307 L308 L309 L310 L311 L312 L313 L314 | L317 L316 L315 | S334 S335 S336 S337 | S345 S344 S343 S342 S341 S340 S339 S338 | L318 L319 S346 S347 S348 S349 S350 S351 L320 L321 S352 S353 S354 S355 S356 L322 L323 | L324 L325 L326 L327 L328 L329 L330 | S357 S358 S359 S360 | S368 S367 S366 S365 S364 S363 S362 S361 bodies 2
body "Solid1"
